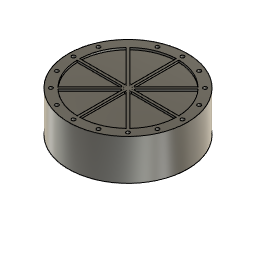
Reaction_Wheel_thick (Autodesk Fusion 360 design; units mm, degrees)
Autodesk Fusion 360 part; units mm, degrees
sketch "스케치1" plane through (0, 0, 0) normal (0, 0, 1) x (1, 0, 0)
  circle A0 centre (0, 0) radius 1.575
  circle A1 centre (0, 0) radius 3.3
  line L0 (0.95, -1.256234) -> (0.95, 1.256234)
  dimension "d1" = 3.15
  dimension "d2" = 6.6
  dimension "d37" = 0.95
  constraint coincident A0.centre A1.centre
  constraint vertical L0
  measures "d1" diameter of A0
  measures "d2" diameter of A1
  measures "d37" distance of A0.centre L0
extrude "돌출1" add sketch "스케치1" along normal blind 30 contours A0 L0 | A1 picked at (1.329433, -0.027761) picked at (2.353535, 1.361247)
sketch "스케치2" plane through (0, 0, 30) normal (0, 0, 1) x (-1, 0, 0)
  circle A0 centre (0, 0) radius 60
  circle A1 centre (0, 0) radius 50
  circle A2 centre (0, 0) radius 3.3
  line L0 (1.310929, -3.028443) -> (1.310929, -49.982812)
  line L1 (-1.310929, -3.028443) -> (-1.310929, -49.982812)
  line L2 (3.068399, -1.214465) -> (36.270152, -34.416218)
  line L3 (1.214465, -3.068399) -> (34.416218, -36.270152)
  line L4 (3.028443, 1.310929) -> (49.982812, 1.310929)
  line L5 (3.028443, -1.310929) -> (49.982812, -1.310929)
  line L6 (1.214465, 3.068399) -> (34.416218, 36.270152)
  line L7 (3.068399, 1.214465) -> (36.270152, 34.416218)
  line L8 (-1.310929, 3.028443) -> (-1.310929, 49.982812)
  line L9 (1.310929, 3.028443) -> (1.310929, 49.982812)
  line L10 (-3.068399, 1.214465) -> (-36.270152, 34.416218)
  line L11 (-1.214465, 3.068399) -> (-34.416218, 36.270152)
  line L12 (-3.028443, -1.310929) -> (-49.982812, -1.310929)
  line L13 (-3.028443, 1.310929) -> (-49.982812, 1.310929)
  line L14 (-1.214465, -3.068399) -> (-34.416218, -36.270152)
  line L15 (-3.068399, -1.214465) -> (-36.270152, -34.416218)
  circle A3 centre (0, 0) radius 5
  dimension "d5" = 120
  dimension "d11" = 100
  dimension "d13" = 360
  dimension "d21" = 10
  constraint coincident A0.centre A1.centre
  constraint concentric A1 A3
  measures "d5" diameter of A0
  measures "d11" diameter of A1
  measures "d21" diameter of A3
extrude "돌출3" add sketch "스케치2" along normal blind 40 contours A0 | A1 L4 L5 A3 | A1 L6 L7 A3 | A2 L2 L4 L5 L7 A3 | L4 L7 A3 | A1 L2 L3 A3 | L2 L5 A3 | A2 L4 L6 L7 L9 A3 | A2 L0 L2 L3 L5 A3 | A1 L8 L9 A3 | L6 L9 A3 | A2 | A1 L0 L1 A3 | L0 L3 A3 | A2 L6 L8 L9 L11 A3 | A2 L0 L1 L3 L14 A3 | A1 L10 L11 A3 | L8 L11 A3 | A1 L14 L15 A3 | L1 L14 A3 | A2 L8 L10 L11 L13 A3 | A2 L1 L12 L14 L15 A3 | A1 L12 L13 A3 | L10 L13 A3 | L12 L15 A3 | A2 L10 L12 L13 L15 A3 picked at (-0.145674, 56.554182) picked at (19.987758, -0.584166) picked at (24.747837, 24.747837) picked at (3.728779, 1.147432) picked at (4.131776, 1.711438) picked at (24.747837, -24.747837) picked at (4.131776, -1.711438) picked at (3.71707, 2.400607) picked at (3.71707, -2.400607) picked at (0, 34.998727) picked at (1.711438, 4.131776) picked at (-0.428905, -0.986319) picked at (0, -34.998727) picked at (1.711438, -4.131776) picked at (-0.93088, 4.325851) picked at (-0.93088, -4.325851) picked at (-24.747837, 24.747837) picked at (-1.711438, 4.131776) picked at (-24.747837, -24.747837) picked at (-1.711438, -4.131776) picked at (-2.400607, 3.71707) picked at (-2.400607, -3.71707) picked at (-34.998727, 0) picked at (-4.131776, 1.711438) picked at (-4.131776, -1.711438) picked at (-4.325851, 0.93088)
sketch "스케치3" plane through (0, 0, 70) normal (0, 0, 1) x (-1, 0, 0)
  circle A0 centre (-55.000001, 0) radius 1.8
  circle A1 centre (-50.813375, -21.047589) radius 1.8
  circle A2 centre (-38.890874, -38.890874) radius 1.8
  circle A3 centre (-21.047589, -50.813375) radius 1.8
  circle A4 centre (0, -55.000001) radius 1.8
  circle A5 centre (21.047589, -50.813375) radius 1.8
  circle A6 centre (38.890874, -38.890874) radius 1.8
  circle A7 centre (50.813375, -21.047589) radius 1.8
  circle A8 centre (55.000001, 0) radius 1.8
  circle A9 centre (50.813375, 21.047589) radius 1.8
  circle A10 centre (38.890874, 38.890874) radius 1.8
  circle A11 centre (21.047589, 50.813375) radius 1.8
  circle A12 centre (0, 55.000001) radius 1.8
  circle A13 centre (-21.047589, 50.813375) radius 1.8
  circle A14 centre (-38.890874, 38.890874) radius 1.8
  circle A15 centre (-50.813375, 21.047589) radius 1.8
  dimension "d33" = 3.6
  dimension "d35" = 360
  measures "d33" diameter of A0
extrude "돌출5" add sketch "스케치2" against normal blind 1 contours A1 L4 L5 A3 | A1 L6 L7 A3 | A2 L2 L4 L5 L7 A3 | L4 L7 A3 | A1 L2 L3 A3 | L2 L5 A3 | A2 L4 L6 L7 L9 A3 | A2 L4 L7 | A2 L0 L2 L3 L5 A3 | A2 L2 L5 | A1 L8 L9 A3 | L6 L9 A3 | A1 L0 L1 A3 | L0 L3 A3 | A2 L6 L8 L9 L11 A3 | A2 L6 L9 | A2 L0 L1 L3 L14 A3 | A2 L0 L3 | A1 L10 L11 A3 | L8 L11 A3 | A1 L14 L15 A3 | L1 L14 A3 | A2 L8 L10 L11 L13 A3 | A2 L8 L11 | A2 L1 L12 L14 L15 A3 | A2 L1 L14 | A1 L12 L13 A3 | L10 L13 A3 | L12 L15 A3 | A2 L10 L12 L13 L15 A3 | A2 L10 L13 | A2 L12 L15 picked at (19.987758, -0.584166) picked at (24.747837, 24.747837) picked at (3.728779, 1.147432) picked at (4.131776, 1.711438) picked at (24.747837, -24.747837) picked at (4.131776, -1.711438) picked at (2.400607, 3.71707) picked at (3.087461, 1.278868) picked at (2.400607, -3.71707) picked at (3.087461, -1.278868) picked at (0, 34.998727) picked at (1.711438, 4.131776) picked at (0, -34.998727) picked at (1.711438, -4.131776) picked at (0.93088, 4.325851) picked at (1.278868, 3.087461) picked at (-0.93088, -4.325851) picked at (1.278868, -3.087461) picked at (-24.747837, 24.747837) picked at (-1.711438, 4.131776) picked at (-24.747837, -24.747837) picked at (-1.711438, -4.131776) picked at (-3.71707, 2.400607) picked at (-1.278868, 3.087461) picked at (-2.400607, -3.71707) picked at (-1.278868, -3.087461) picked at (-34.998727, 0) picked at (-4.131776, 1.711438) picked at (-4.131776, -1.711438) picked at (-4.325851, 0.93088) picked at (-3.087461, 1.278868) picked at (-3.087461, -1.278868)
fillet "모깎기1" radius 10 1 edges at (-3.07668, 1.193331, 29)
extrude "돌출6" add 1 faces at (0.145674, -56.554182, 30) along direction (0, 0, -1) blind 1
extrude "돌출7" add sketch "스케치2" along normal blind 38 contours A1 L4 L7 A3 | A1 L2 L5 A3 | A1 L6 L9 A3 | A1 L0 L3 A3 | A1 L8 L11 A3 | A1 L1 L14 A3 | A1 L10 L13 A3 | A1 L12 L15 A3 picked at (33.850494, 8.536211) picked at (33.850494, -8.536211) picked at (8.536211, 33.850494) picked at (8.536211, -33.850494) picked at (-17.899901, 29.971926) picked at (-8.536211, -33.850494) picked at (-33.850494, 8.536211) picked at (-29.971926, -17.899901)
extrude "돌출8" cut sketch "스케치3" against normal through all contours A0 | A1 | A2 | A3 | A4 | A5 | A7 | A8 | A9 | A10 | A11 | A12 | A13 | A14 | A15 picked at (-54.670745, 0.391437) picked at (-50.91093, -21.296156) picked at (-38.335712, -39.489196) picked at (-21.347589, -52.008974) picked at (-0.3, -56.1956) picked at (21.563287, -51.417646) picked at (50.71582, -21.296156) picked at (55.329257, 0.391437) picked at (50.987742, 21.528452) picked at (39.446035, 38.292551) picked at (21.563287, 50.209105) picked at (0.515698, 54.39573) picked at (-20.531891, 50.209105) picked at (-38.335712, 38.292551) picked at (-50.639008, 21.528452)
